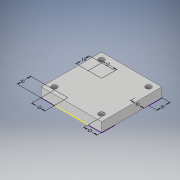
# Autodesk Inventor part: Platte klein
Saved by Autodesk Inventor 2017 (Build 210142000, 142)
## iProperties
Part Number: Platte klein
Material: Generisch
Document SubType Name: Modeling
Designer: pgmadmin
Density: 1 g/cm^3
Appearance: Vorgabe
Author: pgmadmin
Autodesk Inventor part; units mm, degrees
ref_plane "YZ Plane" through (0, 0, 0) normal (1, 0, 0) x (0, 1, 0)
ref_plane "XZ Plane" through (0, 0, 0) normal (0, 1, 0) x (-1, 0, 0)
ref_plane "XY Plane" through (0, 0, 0) normal (0, 0, 1) x (1, 0, 0)
sketch "Skizze1" plane through (0, 0, 0) normal (0, 0, 1) x (1, 0, 0)
  line L0 (-22.5, -22.5) -> (22.5, -22.5)
  line L1 (22.5, -22.5) -> (22.5, 22.5)
  line L2 (22.5, 22.5) -> (-22.5, 22.5)
  line L3 (-22.5, 22.5) -> (-22.5, -22.5)
  line L4 (-22.5, -22.5) -> (22.5, 22.5) construction
  line L5 (22.5, -22.5) -> (-22.5, 22.5) construction
  point P0 (0, 0)
  dimension "d0" = 45
  dimension "d1" = 45
  constraints: 12 end point, 2 midpoint, 2 parallel, 1 horizontal, 1 perpendicular
  measures "d0" distance of L2.end L1.end
  measures "d1" distance of L1.end L0.end
extrude "Extrusion1" add sketch "Skizze1" along normal blind 7
sketch "Skizze2" plane through (0, 0, 0) normal (0, 0, -1) x (-1, 0, 0)
  line L0 (-22.5, -22.5) -> (-22.5, 22.5) projected
  line L1 (-22.5, 22.5) -> (22.5, 22.5) projected
  line L2 (22.5, 22.5) -> (22.5, -22.5) projected
  line L3 (22.5, -22.5) -> (-22.5, -22.5) projected
  point P0 (0, 0)
  point P1 (-17.5, 17.5)
  point P2 (17.5, 17.5)
  point P3 (17.5, -17.5)
  point P4 (-17.5, -17.5)
  dimension "d4" = 5
  dimension "d5" = 5
  dimension "d6" = 5
  dimension "d7" = 5
  dimension "d8" = 5
  dimension "d9" = 5
  dimension "d12" = 5
  dimension "d13" = 5
  measures "d4" distance from line of L0 point (-17.5, 17.5)
  measures "d5" distance from line of point (-17.5, 17.5) L1
  measures "d6" distance from line of L1 point (17.5, 17.5)
  measures "d7" distance from line of L2 point (17.5, 17.5)
  measures "d8" distance from line of L2 point (17.5, -17.5)
  measures "d9" distance from line of L3 point (17.5, -17.5)
  measures "d12" distance from line of L0 point (-17.5, -17.5)
  measures "d13" distance from line of L3 point (-17.5, -17.5)
hole "Bohrung1" at (17.5, 17.5, 0) at (-17.5, 17.5, 0) at (-17.5, -17.5, 0) at (17.5, -17.5, 0) direction (0, 0, 1) diameter 4 end through all
sketch "Skizze3" plane through (0, 0, 0) normal (0, 0, -1) x (-1, 0, 0)
  line L0 (-22.5, 22.5) -> (22.5, 22.5) projected
  line L1 (-22.5, 22.5) -> (-12.5, 22.5)
  line L2 (-12.5, 22.5) -> (-12.5, 12.5)
  line L3 (-12.5, 12.5) -> (-22.5, 12.5)
  line L4 (-22.5, 12.5) -> (-22.5, 22.5)
  line L5 (22.5, 22.5) -> (12.5, 22.5)
  line L6 (12.5, 22.5) -> (12.5, 12.5)
  line L7 (12.5, 12.5) -> (22.5, 12.5)
  line L8 (22.5, 12.5) -> (22.5, 22.5)
  line L9 (22.5, 22.5) -> (22.5, -22.5) projected
  line L10 (22.5, -22.5) -> (12.5, -22.5)
  line L11 (12.5, -22.5) -> (12.5, -12.5)
  line L12 (12.5, -12.5) -> (22.5, -12.5)
  line L13 (22.5, -12.5) -> (22.5, -22.5)
  line L14 (22.5, -22.5) -> (-22.5, -22.5) projected
  line L15 (-22.5, -22.5) -> (-12.5, -22.5)
  line L16 (-12.5, -22.5) -> (-12.5, -12.5)
  line L17 (-12.5, -12.5) -> (-22.5, -12.5)
  line L18 (-22.5, -12.5) -> (-22.5, -22.5)
  point P0 (0, 0)
  dimension "d21" = 10
  dimension "d22" = 10
  dimension "d23" = 10
  dimension "d24" = 10
  dimension "d25" = 10
  dimension "d26" = 10
  dimension "d27" = 10
  constraints: 32 end point, 8 parallel, 4 horizontal, 4 perpendicular, 1 point on line
  measures "d21" distance of L2.end L3.end
  measures "d22" distance of L3.end L0.start
  measures "d23" distance of L5.end L6.end
  measures "d24" distance of L6.end L7.end
  measures "d25" distance of L11.end L12.end
  measures "d26" distance of L10.end L11.end
  measures "d27" distance of L16.end L17.end
